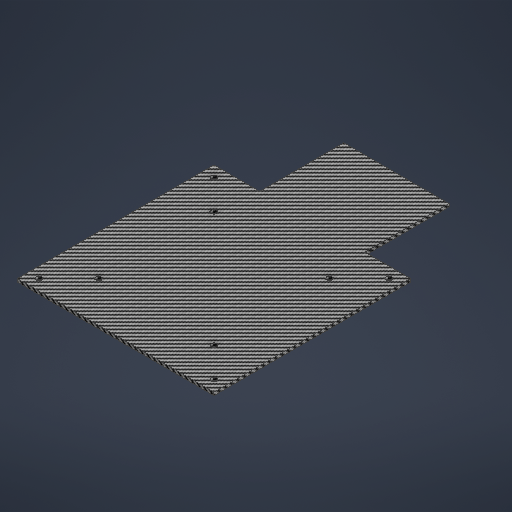
# Autodesk Inventor part: swtc1
Saved by Autodesk Inventor 2026.1 (Build 301233020, 233B)
## iProperties
Created: 2025-09-23
Part Number: swtc1
Material: Polímero reforzado con fibra de carbono
Document SubType Name: Modeling
Designer: rodri
Density: 1.43 g/cm^3
Appearance: Fibra de carbono
Author: rodri
Autodesk Inventor part; units mm, degrees
ref_plane "YZ Plane" through (0, 0, 0) normal (1, 0, 0) x (0, 1, 0)
ref_plane "XZ Plane" through (0, 0, 0) normal (0, 1, 0) x (-1, 0, 0)
ref_plane "XY Plane" through (0, 0, 0) normal (0, 0, 1) x (1, 0, 0)
sketch "Boceto1" plane through (0, 0, 0) normal (0, 1, 0) x (-1, 0, 0)
  line L0 (-58.5, -58.5) -> (58.5, -58.5)
  line L1 (58.5, -58.5) -> (58.5, 58.5)
  line L2 (58.5, 58.5) -> (-58.5, 58.5)
  line L3 (-58.5, 58.5) -> (-58.5, -58.5)
  line L4 (-58.5, -58.5) -> (58.5, 58.5) construction
  line L5 (58.5, -58.5) -> (-58.5, 58.5) construction
  line L6 (-52, 52) -> (52, 52) construction
  line L7 (52, 52) -> (52, -52) construction
  line L8 (52, -52) -> (-52, -52) construction
  line L9 (-52, -52) -> (-52, 52) construction
  line L10 (-52, 52) -> (52, -52) construction
  line L11 (52, 52) -> (-52, -52) construction
  line L12 (34.3223, 34.3223) -> (-34.3223, 34.3223) construction
  line L13 (-34.3223, 34.3223) -> (-34.3223, -34.3223) construction
  line L14 (-34.3223, -34.3223) -> (34.3223, -34.3223) construction
  line L15 (34.3223, -34.3223) -> (34.3223, 34.3223) construction
  line L16 (34.3223, 34.3223) -> (-34.3223, -34.3223) construction
  line L17 (-34.3223, 34.3223) -> (34.3223, -34.3223) construction
  line L18 (0, -58.5) -> (0, -108.5) construction
  line L19 (31.3, -58.5) -> (-31.3, -58.5)
  line L20 (-31.3, -58.5) -> (-31.3, -108.5)
  line L21 (-31.3, -108.5) -> (31.3, -108.5)
  line L22 (31.3, -108.5) -> (31.3, -58.5)
  line L23 (31.3, -58.5) -> (-31.3, -108.5) construction
  line L24 (-31.3, -58.5) -> (31.3, -108.5) construction
  point P0 (0, 0)
  point P1 (0, -83.5)
  dimension "d0" = 117
  dimension "d1" = 117
  dimension "d2" = 104
  dimension "d3" = 25
  dimension "d4" = 50
  dimension "d5" = 62.6
  constraints: 50 end point, 10 midpoint, 8 parallel, 4 horizontal, 4 perpendicular, 2 point on line, 1 vertical
  measures "d0" distance of L1.end L2.end
  measures "d1" distance of L0.end L1.end
  measures "d2" distance of L7.end L8.end
  measures "d3" distance of L8.end L13.end
  measures "d4" distance of L18.start L18.end
  measures "d5" distance of L20.end L21.end
extrude "Extrusión1" add sketch "Boceto1" against normal blind 1.8
hole "Agujero1" at (-52, 0, -52) at (-34.3223, 0, -34.3223) at (-52, 0, 52) at (-34.3223, 0, 34.3223) at (52, 0, 52) at (34.3223, 0, 34.3223) at (34.3223, 0, -34.3223) at (52, 0, -52) direction (0, -1, 0) diameter 3.4 end through all clearance for "Tornillo para maquinaria de cabeza plana" size "M3" standard "Perfil M métrico ANSI"
